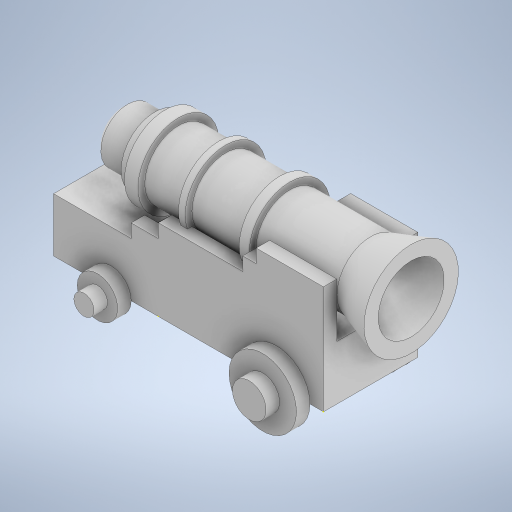
# Autodesk Inventor part: Cannon
Saved by Autodesk Inventor 2024.1 (Build 281209000, 209)
## iProperties
Created: 2023-10-24
Part Number: Cannon
Material: Generic
Document SubType Name: Modeling
Designer: luvag
Density: 1 g/cm^3
Appearance: Default
Author: luvag
Autodesk Inventor part; units mm, degrees
sketch "Sketch1" plane through (0, 0, 0) normal (0, 0, 1) x (1, 0, 0)
  line L0 (0, 0) -> (2000, 0)
  line L1 (2000, 0) -> (2000, 601.8912)
  line L2 (1401.6262, 601.8912) -> (776.6262, 601.8912)
  line L3 (776.6262, 601.8912) -> (776.6262, 600)
  line L4 (776.6262, 600) -> (775, 600)
  line L5 (775, 600) -> (775, 500)
  line L6 (775, 500) -> (575, 500)
  line L7 (575, 500) -> (575, 400)
  line L8 (575, 400) -> (0, 400)
  line L9 (0, 400) -> (0, 0)
  line L10 (1401.6262, 601.8912) -> (1401.6262, 701.8912)
  line L11 (1401.6262, 701.8912) -> (1501.6262, 701.8912)
  line L12 (1501.6262, 701.8912) -> (1501.6262, 801.8912)
  line L13 (1501.6262, 801.8912) -> (2000, 801.8912)
  line L14 (2000, 801.8912) -> (2000, 601.8912)
  dimension "d0" = 2000
  dimension "d1" = 400
  dimension "d2" = 575
  dimension "d3" = 100
  dimension "d4" = 200
  dimension "d5" = 100
  dimension "d6" = 625
  dimension "d7" = 100
  dimension "d8" = 100
  dimension "d9" = 100
  constraints: 30 end point, 7 perpendicular, 3 parallel, 2 horizontal, 1 vertical
  measures "d0" distance of L0.start L0.end
  measures "d1" distance of L8.end L0.start
  measures "d2" distance of L7.end L8.end
  measures "d3" distance of L6.end L7.end
  measures "d4" distance of L5.end L6.end
  measures "d5" distance of L4.end L5.end
  measures "d6" distance of L2.start L2.end
  measures "d7" distance of L2.start L10.end
  measures "d8" distance of L11.end L12.end
  measures "d9" distance of L10.end L11.end
extrude "Extrusion1" add sketch "Sketch1" against normal blind 700
sketch "Sketch2" plane through (2000, 0, 0) normal (1, 0, 0) x (0, 0, -1)
  line L0 (0, 801.8912) -> (100, 801.8912)
  line L1 (100, 801.8912) -> (100, 401.8912)
  line L2 (100, 401.8912) -> (603.8012, 401.8912)
  arc A0 (603.8012, 401.8912) -> (600, 801.8912) centre (-20444.0043, 401.8912) ccw
  line L3 (0, 801.8912) -> (700, 801.8912) projected
  line L4 (600, 801.8912) -> (700, 801.8912)
  point P0 (0, 0)
  dimension "d12" = 100
  dimension "d13" = 100
  dimension "d14" = 400
  constraints: 8 end point, 2 point on circle, 1 centre point, 1 horizontal, 1 perpendicular, 1 point on line
  measures "d12" distance of L0.start L0.end
  measures "d13" distance of L4.start L3.end
  measures "d14" distance of L0.end L1.end
extrude "Extrusion2" cut sketch "Sketch2" against normal blind 10000
sketch "Sketch3" plane through (2000, 0, 0) normal (1, 0, 0) x (0, 0, -1)
  line L0 (100, 701.8912) -> (100, 601.8912) projected
  line L1 (100, 700) -> (350, 700)
  line L2 (100, 401.8912) -> (100, 801.8912) projected
  line L3 (100, 401.8912) -> (350, 400)
  line L4 (0, 400) -> (700, 400) projected
  line L5 (350, 700) -> (350, 400)
  line L6 (603.8012, 401.8912) -> (100, 401.8912) projected
  circle A0 centre (350, 700) radius 250
  point P0 (0, 0)
  dimension "d17" = 300
  dimension "d18" = 250
  dimension "d22" = 500
  constraints: 6 end point, 1 centre point, 1 coincident, 1 horizontal, 1 midpoint, 1 parallel, 1 perpendicular, 1 point on line
  measures "d17" distance of L1.end L3.end
  measures "d18" distance of L1.start L1.end
  measures "d22" diameter of A0
extrude "Extrusion3" [suppressed]
extrude "Extrusion4" add sketch "Sketch3" against normal blind 1600 contours A0 L5 L1 | L1 L5 A0
ref_plane "Work Plane1" through (475, 700, -350) normal (-1, 0, 0) x (0, 0, 1)
sketch "Sketch4" plane through (475, 700, -350) normal (-1, 0, 0) x (0, 0, 1)
  circle A0 centre (0, 0) radius 300
  point P0 (350, -700)
  dimension "d26" = 600
  constraints: 1 centre point
  measures "d26" diameter of A0
extrude "Extrusion5" add sketch "Sketch4" against normal blind 100
ref_plane "Work Plane2" through (775, 700, -350) normal (-1, 0, 0) x (0, 0, 1)
sketch "Sketch5" plane through (775, 700, -350) normal (-1, 0, 0) x (0, 0, 1)
  point P0 (350, -700)
sketch "Sketch6" plane through (775, 700, -350) normal (-1, 0, 0) x (0, 0, 1)
  point P0 (350, -700)
ref_plane "Work Plane4" through (875, 700, -350) normal (-1, 0, 0) x (0, 0, 1)
sketch "Sketch7" plane through (875, 700, -350) normal (-1, 0, 0) x (0, 0, 1)
  circle A0 centre (0, 0) radius 300
  point P0 (350, -700)
  constraints: 1 centre point
extrude "Extrusion6" add sketch "Sketch7" against normal blind 50
ref_plane "Work Plane5" through (1325, 700, -350) normal (-1, 0, 0) x (0, 0, 1)
sketch "Sketch8" plane through (1325, 700, -350) normal (-1, 0, 0) x (0, 0, 1)
  circle A0 centre (0, 0) radius 300
  point P0 (350, -700)
  constraints: 1 centre point
extrude "Extrusion7" add sketch "Sketch8" against normal blind 75
ref_plane "Work Plane6" through (0, 0, -350) normal (0, 0, 1) x (1, 0, 0)
sketch "Sketch9" plane through (0, 0, -350) normal (0, 0, 1) x (1, 0, 0)
  point P0 (0, 0)
sketch "Sketch10" plane through (0, 0, -350) normal (0, 0, 1) x (1, 0, 0)
  line L0 (2000, 801.8912) -> (2000, 0) projected
  line L1 (2000, 450) -> (2000, 950) projected
  line L2 (2300, 1050) -> (2000, 950)
  line L3 (2000, 700) -> (2000, 801.8912)
  line L4 (2000, 700) -> (1401.6262, 700) projected
  line L5 (2000, 700) -> (2300, 700)
  line L6 (2300, 700) -> (2300, 1050)
  line L7 (2192.8359, 1014.2786) -> (2224.4587, 919.4103)
  line L8 (2300, 1050) -> (2300, 996.3475)
  line L9 (2250.0255, 1033.3418) -> (2281.6483, 938.4735)
  line L10 (2300, 944.5907) -> (2281.6483, 938.4735)
  line L11 (2224.4587, 919.4103) -> (2281.6483, 938.4735)
  line L12 (2281.6483, 938.4735) -> (2000, 844.5907)
  point P0 (0, 0)
  dimension "d39" = 350
  dimension "d40" = 300
  dimension "d41" = 100
  dimension "d42" = 100
  constraints: 20 end point, 5 point on line, 2 collinear, 2 perpendicular, 1 horizontal, 1 parallel
  measures "d39" distance of L5.end L2.start
  measures "d40" distance of L3.start L5.end
  measures "d41" distance of L9.start L9.end
  measures "d42" distance of L7.start L7.end
sketch "Sketch11" plane through (0, 0, -350) normal (0, 0, 1) x (1, 0, 0)
  point P0 (0, 0)
revolve "Revolution1" add sketch "Sketch10" angle 360 about axis through (2000, 700, -350) along (1, 0, 0) contours L1 L2 L7 L12 | L7 L2 L9 L11 | L10 L9 L2 L6
sketch "Sketch12" plane through (0, 0, -350) normal (0, 0, 1) x (1, 0, 0)
  line L0 (400, 950) -> (400, 450) projected
  line L1 (400, 950) -> (400, 700)
  line L2 (400, 700) -> (200, 700)
  line L3 (200, 700) -> (200, 900)
  line L4 (200, 900) -> (400, 900)
  line L5 (200, 700) -> (100, 700)
  arc A0 (200, 900) -> (100, 700) centre (366.9965, 691.5017) ccw
  point P0 (0, 0)
  dimension "d44" = 200
  dimension "d45" = 200
  dimension "d46" = 100
  constraints: 10 end point, 2 point on circle, 1 centre point, 1 midpoint, 1 point on line
  measures "d44" distance of L1.end L2.end
  measures "d45" distance of L2.end L3.end
  measures "d46" distance of L2.end L5.end
revolve "Revolution2" add sketch "Sketch12" angle 360 about axis through (400, 700, -350) along (-1, 0, 0)
sketch "Sketch13" plane through (2000, 700, -350) normal (1, 0, 0) x (0, 0, -1)
  point P0 (-350, -700)
sketch "Sketch14" plane through (2000, 700, -350) normal (1, 0, 0) x (0, 0, -1)
  circle A0 centre (0, 0) radius 144.5907 projected
  circle A1 centre (0, 0) radius 144.5907
  point P0 (-350, -700)
  constraints: 1 centre point, 1 coincident
extrude "Extrusion8" cut sketch "Sketch14" against normal blind 1800
sketch "Sketch15" plane through (0, 0, -700) normal (0, 0, -1) x (-1, 0, 0)
  line L0 (0, 0) -> (-2000, 0) projected
  line L1 (0, 0) -> (-425, 0)
  circle A0 centre (-425, 0) radius 150
  line L2 (-2000, 0) -> (-1650, 0)
  circle A1 centre (-1650, 0) radius 250
  dimension "d50" = 425
  dimension "d51" = 300
  dimension "d52" = 350
  dimension "d53" = 500
  constraints: 4 end point, 2 centre point, 2 coincident, 2 point on line
  measures "d50" distance of L0.start L1.end
  measures "d51" diameter of A0
  measures "d52" distance of L0.end L2.end
  measures "d53" diameter of A1
extrude "Extrusion9" add sketch "Sketch15" along normal blind 100
sketch "Sketch16" plane through (1650, 0, -800) normal (0, 0, -1) x (-1, 0, 0)
  arc A0 (1075, 0) -> (1375, 0) centre (1225, 0) ccw projected
  circle A1 centre (1225, 0) radius 75
  arc A2 (-250, 0) -> (250, 0) centre (0, 0) ccw projected
  circle A3 centre (0, 0) radius 125
  point P0 (1650, 0)
  dimension "d56" = 150
  dimension "d57" = 250
  constraints: 2 centre point, 2 coincident
  measures "d56" diameter of A1
  measures "d57" diameter of A3
extrude "Extrusion10" add sketch "Sketch16" along normal blind 100
mirror "Mirror1" about plane through (0, 0, -350) normal (0, 0, 1) of "Extrusion9", "Extrusion10"
body "Solid1"
